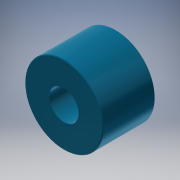
# Autodesk Inventor part: 13-0004
Saved by Autodesk Inventor 2017.1 (Build 211199000, 199)
## iProperties
Category: Matrix
Company: Autodesk Inc.
Created: 2014-11-30
Part Number: 13-0004
Material: Polystyrene, High Impact
Document SubType Name: Modeling
Designer: Matrix
Density: 1.022 g/cm^3
Appearance: Sky Blue Dark
Catalog Web Link: http://matrixrobotics.com/
Vendor: Matrix
Author: Autodesk Inc.
Autodesk Inventor part; units mm, degrees
ref_plane "YZ Plane" through (0, 0, 0) normal (1, 0, 0) x (0, 1, 0)
ref_plane "XZ Plane" through (0, 0, 0) normal (0, 1, 0) x (-1, 0, 0)
ref_plane "XY Plane" through (0, 0, 0) normal (0, 0, 1) x (1, 0, 0)
sketch "Sketch1" plane through (0, 0, 0) normal (0, 1, 0) x (-1, 0, 0)
  circle A0 centre (0, 0) radius 6
  dimension "d0" = 12
  constraints: 1 centre point, 1 coincident
  measures "d0" diameter of A0
extrude "Extrusion1" add sketch "Sketch1" against normal blind 8
chamfer "Chamfer1" distance 0.1 angle 45 2 edges at (6, -8, 0) (6, 0, 0)
sketch "Sketch2" plane through (0, -8, 0) normal (0, -1, 0) x (1, 0, 0)
  point P0 (0, 0)
hole "Hole1" at (0, -8, 0) direction (0, 1, 0) diameter 4.5 end through all
body "Solid1"
